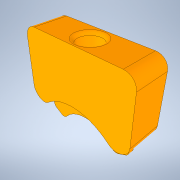
# Autodesk Inventor part: Бегунок
Saved by Autodesk Inventor 2021.1 (Build 251245010, 245A)
## iProperties
Created: 2026-04-16
Part Number: Бегунок
Material: Типовые
Document SubType Name: Modeling
Designer: Андрей Тарасов
Density: 1 g/cm^3
Appearance: По умолчанию
Author: Андрей Тарасов
Autodesk Inventor part; units mm, degrees
ref_plane "YZ Plane" through (0, 0, 0) normal (1, 0, 0) x (0, 1, 0)
ref_plane "XZ Plane" through (0, 0, 0) normal (0, 1, 0) x (-1, 0, 0)
sketch "Эскиз1" plane through (0, 0, 0) normal (0, 0, 1) x (1, 0, 0)
  line L0 (0, 0) -> (-14.5, 0)
  line L1 (14.5, 0) -> (0, 0)
  line L2 (0, -16) -> (0, 26) construction
  line L3 (-20.3, 0) -> (20.3, 0) construction
  line L4 (-10, 0) -> (-10, 20)
  line L5 (10, 0) -> (10, 20)
  line L6 (-10, 20) -> (10, 20)
  line L7 (-10, 8.391) -> (0, 0)
  line L8 (0, 0) -> (10, 8.391)
  circle A0 centre (0, 0) radius 10
  point P0 (-7.6604, 6.4279)
  point P1 (7.6604, 6.4279)
  dimension "d2" = 180
  dimension "d3" = 90
  dimension "d26" = 20
  dimension "d47" = 40
  dimension "d48" = 40
  dimension "d49" = 20
  constraints: 15 end point, 4 point on line, 2 coincident, 2 tangent, 2 vertical, 1 centre point, 1 horizontal
  measures "d2" angle of L1 L0
  measures "d3" angle of L2 L0
  measures "d26" distance between parallel lines of L6 L3
  measures "d47" angle of L3 L7
  measures "d48" angle of L3 L8
  measures "d49" diameter of A0
extrude "Выдавливание1" add sketch "Эскиз1" along normal blind 6 contours L7 L4 L6 L5 L8 A0
sketch "Эскиз5" plane through (-10, 20, 0) normal (0, 1, 0) x (1, 0, 0)
  line L0 (10, 0) -> (10, -6) construction
  line L1 (20, -6) -> (0, -6) projected
  circle A0 centre (10, -3) radius 2.1
  dimension "d50" = 4.2
  constraints: 2 end point, 2 midpoint, 1 centre point
  measures "d50" diameter of A0
extrude "Выдавливание3" cut sketch "Эскиз5" against normal blind 8
sketch "Эскиз6" plane through (0, 12, 3) normal (0, 1, 0) x (1, 0, 0)
  circle A0 centre (0, 0) radius 2.1 projected
  circle A1 centre (0, 0) radius 1
  line L0 (0, -1) -> (0, 1)
  point P0 (0, 3)
  dimension "d53" = 2
  constraints: 2 end point, 2 point on circle, 1 centre point, 1 coincident, 1 midpoint, 1 vertical
  measures "d53" diameter of A1
revolve "Вращение4" cut sketch "Эскиз6" angle 360 about axis through (0, 12, 4) along (0, 0, -1) picked at (0.2078, 0.2606) contours A1 L0
fillet "Сопряжение6" radius 0.6 4 edges at (-2.1, 20, 3) (-2.1, 12, 3) (1, 12, 3) (-1, 12, 3)
fillet "Сопряжение6" radius 2 6 edges at (-7.6604, 6.4279, 3) (7.6604, 6.4279, 3) (-10, 8.391, 3) (10, 8.391, 3) (-10, 20, 3) (10, 20, 3)
ref_plane "РабПлоскость3" through (0, 0, 3) normal (0, 0, 1) x (1, 0, 0)
sketch "Эскиз7" plane through (0, 0, 3) normal (0, 0, 1) x (1, 0, 0)
  circle A0 centre (0, 0) radius 6.5
  circle A1 centre (0, 0) radius 10
  arc A2 (6.482, 7.6147) -> (-6.482, 7.6147) centre (0, 0) ccw projected
  line L0 (0, 0) -> (-8.6603, 5)
  line L1 (0, 0) -> (8.6603, 5)
  line L2 (-14, 0) -> (14, 0) construction
  point P0 (5.6292, 3.25)
  point P1 (-5.6292, 3.25)
  dimension "d57" = 13
  dimension "d61" = 30
  dimension "d62" = 30
  constraints: 4 end point, 2 centre point, 2 coincident, 2 point on circle, 1 concentric
  measures "d57" diameter of A0
  measures "d61" angle of L2 L0
  measures "d62" angle of L2 L1
extrude "Выдавливание4" add sketch "Эскиз7" along normal mid plane 1 contours A0 L0 A1 L1 picked at (4.8613, 7.3201)
fillet "Сопряжение7" radius 1 4 edges at (-5.6292, 3.25, 3) (5.6292, 3.25, 3) (8.6603, 5, 3) (-8.6603, 5, 3)
equation "\"d3\" = 0.5 * d2"
equation "\"d48\" = d47"
